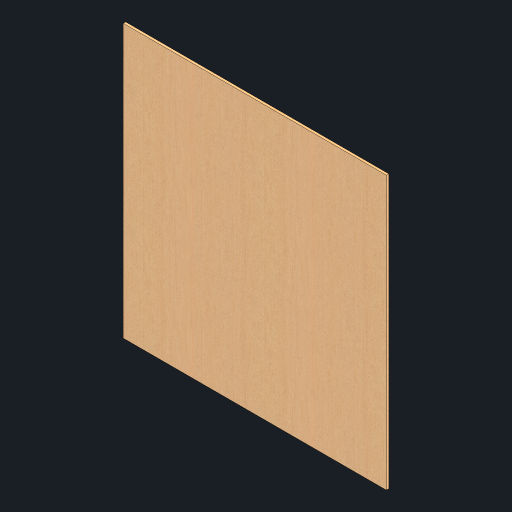
# Autodesk Inventor part: 570x610 패널
Saved by Autodesk Inventor 2024.1 (Build 281209000, 209)
## iProperties
Created: 2024-01-12
Part Number: 570x610 패널
Material: 일반
Document SubType Name: Modeling
Designer: KBU
Density: 1 g/cm^3
Appearance: 기본값
Author: KBU
Autodesk Inventor part; units mm, degrees
ref_plane "YZ Plane" through (0, 0, 0) normal (1, 0, 0) x (0, 1, 0)
ref_plane "XZ Plane" through (0, 0, 0) normal (0, 1, 0) x (-1, 0, 0)
ref_plane "XY Plane" through (0, 0, 0) normal (0, 0, 1) x (1, 0, 0)
sketch "스케치1" plane through (0, 0, 0) normal (0, 0, 1) x (1, 0, 0)
  line L0 (-275, -285) -> (275, -285)
  line L1 (275, -285) -> (275, 285)
  line L2 (275, 285) -> (-275, 285)
  line L3 (-275, 285) -> (-275, -285)
  line L4 (-275, -285) -> (275, 285) construction
  line L5 (275, -285) -> (-275, 285) construction
  point P0 (0, 0)
  dimension "d0" = 550
  dimension "d1" = 570
  constraints: 12 end point, 2 midpoint, 2 parallel, 1 horizontal, 1 perpendicular
  measures "d0" distance of L1.end L2.end
  measures "d1" distance of L0.end L1.end
extrude "돌출1" add sketch "스케치1" along normal blind 5
